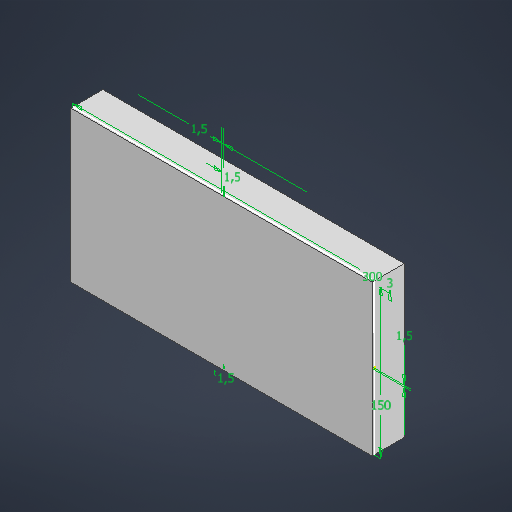
# Autodesk Inventor part: nsabo
Saved by Autodesk Inventor 2026.2 (Build 302298010, 298A)
## iProperties
Created: 2026-04-26
Part Number: nsabo
Material: Genérico
Document SubType Name: Modeling
Designer: Lucas David
Density: 1 g/cm^3
Appearance: Padrão
Author: Lucas David
Autodesk Inventor part; units mm, degrees
ref_plane "YZ Plane" through (0, 0, 0) normal (1, 0, 0) x (0, 1, 0)
ref_plane "XZ Plane" through (0, 0, 0) normal (0, 1, 0) x (-1, 0, 0)
ref_plane "XY Plane" through (0, 0, 0) normal (0, 0, 1) x (1, 0, 0)
sketch "Esboço1" plane through (0, 0, 0) normal (0, 0, 1) x (1, 0, 0)
  line L0 (-150, -75) -> (150, -75)
  line L1 (150, -75) -> (150, 75)
  line L2 (150, 75) -> (-150, 75)
  line L3 (-150, 75) -> (-150, -75)
  line L4 (-150, -75) -> (150, 75) construction
  line L5 (-147, 72) -> (147, 72)
  line L6 (147, 72) -> (147, -72)
  line L7 (147, -72) -> (-147, -72)
  line L8 (-147, -72) -> (-147, 72)
  line L9 (0, 72) -> (0, 0) construction
  line L10 (147, 0) -> (0, 0) construction
  line L11 (1.5, 72) -> (1.5, 1.5)
  line L12 (1.5, 1.5) -> (147, 1.5)
  line L13 (0, 0) -> (0, -72) construction
  line L14 (147, -1.5) -> (1.5, -1.5)
  line L15 (1.5, -1.5) -> (1.5, -72)
  line L16 (150, -75) -> (144, -72) construction
  line L17 (0, 0) -> (-150, 75) construction
  line L18 (-1.5, 72) -> (-1.5, 0)
  line L19 (-1.5, 0) -> (-1.5, -72)
  dimension "d0" = 150
  dimension "d1" = 300
  dimension "d2" = 3
  dimension "d3" = 1.5
  dimension "d5" = 1.5
  dimension "d6" = 1.5
  dimension "d7" = 1.5
  constraints: 40 end point, 6 parallel, 4 midpoint, 4 perpendicular, 1 horizontal, 1 point on line, 1 vertical, 5 other
  measures "d0" distance between parallel lines of L0 L2
  measures "d1" distance between parallel lines of L1 L3
  measures "d2" distance between parallel lines of L2 L5
  measures "d3" distance between parallel lines of L9 L11
  measures "d5" distance between parallel lines of L10 L14
  measures "d6" distance between parallel lines of L13 L15
  measures "d7" distance between parallel lines of L18 L9
extrude "Extrusão1" add sketch "Esboço1" along normal blind 2 contours L3 L2 L1 L0 | L5 L18 L19 L7 L8 | L5 L11 L12 L6 L14 L15 L7 L19 L18 | L5 L6 L12 L11 | L15 L14 L6 L7
extrude "Extrusão2" add sketch "Esboço1" against normal blind 30 contours L3 L2 L1 L0 | L5 L11 L12 L6 L14 L15 L7 L19 L18
sketch "Esboço2" plane through (150, -75, 2) normal (1, 0, 0) x (0, 0, -1)
  point P0 (2, 75)
